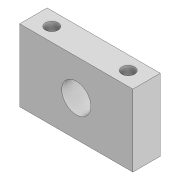
# Autodesk Inventor part: T8_NUT_HOUSING
Saved by Autodesk Inventor 2022 (Build 260153000, 153)
## iProperties
Created: 2021-04-23
Part Number: T8_NUT_HOUSING
Material: Generic
Document SubType Name: Modeling
Designer: nnico
Density: 1 g/cm^3
Appearance: Default
Author: nnico
Autodesk Inventor part; units mm, degrees
ref_plane "YZ Plane" through (0, 0, 0) normal (1, 0, 0) x (0, 1, 0)
ref_plane "XZ Plane" through (0, 0, 0) normal (0, 1, 0) x (-1, 0, 0)
ref_plane "XY Plane" through (0, 0, 0) normal (0, 0, 1) x (1, 0, 0)
sketch "Sketch1" plane through (0, 0, 0) normal (0, 1, 0) x (-1, 0, 0)
  line L0 (20, -4.85) -> (-20, -4.85)
  line L1 (-20, -4.85) -> (-20, 4.85)
  line L2 (-20, 4.85) -> (20, 4.85)
  line L3 (20, 4.85) -> (20, -4.85)
  line L4 (0, -4.85) -> (0, 4.85) construction
  line L5 (20, 0) -> (-20, 0) construction
  circle A0 centre (13.5, 0) radius 2.25
  circle A1 centre (-13.5, 0) radius 2.25
  point P0 (0, 0)
  point P1 (0, 0)
  dimension "d0" = 40
  dimension "d1" = 9.7
  dimension "d2" = 4.5
  dimension "d3" = 27
  constraints: 12 end point, 5 midpoint, 2 centre point, 2 parallel, 1 coincident, 1 horizontal, 1 perpendicular, 1 point on line, 1 symmetric about line, 1 other
  measures "d0" distance of L1.end L2.end
  measures "d1" distance of L0.end L1.end
  measures "d2" diameter of A0
  measures "d3" diameter of A0.centre L4
extrude "Extrusion1" add sketch "Sketch1" along normal blind 25.4
sketch "Sketch2" plane through (-20, 0, 4.85) normal (0, 0, 1) x (1, 0, 0)
  line L0 (0, 0) -> (0, 25.4) construction
  line L1 (0, 12.7) -> (40, 12.7) construction
  line L2 (40, 0) -> (40, 25.4) construction
  line L3 (20, 0) -> (20, 25.4) construction
  line L4 (0, 25.4) -> (40, 25.4) construction
  circle A0 centre (20, 12.7) radius 5.15
  dimension "d6" = 10.3
  constraints: 4 end point, 4 midpoint, 1 centre point
  measures "d6" diameter of A0
extrude "Extrusion2" cut sketch "Sketch2" against normal through all
body "Solid1"
